Autodesk Fusion 360 part; units mm, degrees
note: some values were not read from the file. Chosen so that the rebuilt part matches the saved one: a direction. Set by a fixed rule: which sketch regions a step uses.
(part 4 of 6)
sketch "Sketch6" plane through (-0.4707, 0.1724, 6) normal (0, 0, 1) x (-0.999921, 0.012548, 0)
  arc A0 (-25.3686, -35.2487) -> (-25.5248, -36.2599) centre (-13.5, -37.5997) ccw
  arc A1 (-25.6343, -36.3483) -> (-25.5248, -36.2599) centre (-25.6242, -36.2488) ccw
  line L0 (-25.6343, -36.3483) -> (-26.119, -36.299)
  spline S0 degree 5 poles (-26.119, -36.299) (-26.1246, -36.2984) (-26.1359, -36.2974) (-26.1528, -36.2963) (-26.1754, -36.2957) (-26.2037, -36.2959) (-26.2321, -36.297) (-26.2605, -36.2985) (-26.2889, -36.3004) (-26.3173, -36.3024) (-26.3458, -36.3046) (-26.3743, -36.307) (-26.4028, -36.3098) (-26.4313, -36.313) (-26.4598, -36.3165) (-26.4883, -36.3204) (-26.5168, -36.3246) (-26.5454, -36.3291) (-26.5739, -36.3338) (-26.6025, -36.3387) (-26.6311, -36.3438) (-26.6596, -36.3492) (-26.6882, -36.3548) (-26.7168, -36.3606) (-26.7453, -36.3667) (-26.7739, -36.3729) (-26.8025, -36.3795) (-26.8311, -36.3862) (-26.8596, -36.3931) (-26.8882, -36.4002) (-26.9168, -36.4076) (-26.9453, -36.4151) (-26.9739, -36.4228) (-27.0024, -36.4307) (-27.031, -36.4388) (-27.0595, -36.4471) (-27.088, -36.4555) (-27.1166, -36.4642) (-27.1451, -36.473) (-27.1736, -36.482) (-27.2021, -36.4912) (-27.2306, -36.5006) (-27.2591, -36.5101) (-27.2875, -36.5198) (-27.316, -36.5297) (-27.3444, -36.5398) (-27.3729, -36.55) (-27.4013, -36.5604) (-27.4297, -36.5709) (-27.4581, -36.5816) (-27.4865, -36.5925) (-27.5149, -36.6035) (-27.5432, -36.6147) (-27.5716, -36.6261) (-27.5999, -36.6376) (-27.6282, -36.6493) (-27.6565, -36.6611) (-27.6848, -36.673) (-27.7131, -36.6852) (-27.7413, -36.6975) (-27.7696, -36.7099) (-27.7978, -36.7225) (-27.826, -36.7352) (-27.8541, -36.7481) (-27.8823, -36.7611) (-27.9104, -36.7743) (-27.9386, -36.7876) (-27.9666, -36.801) (-27.9947, -36.8146) (-28.0228, -36.8284) (-28.0508, -36.8423) (-28.0732, -36.8535) (-28.09, -36.862) (-28.1012, -36.8677) (-28.1068, -36.8705) knots 0 0 0 0 0 0 0.01428571 0.02857143 0.04285714 0.05714286 0.07142857 0.08571429 0.1 0.11428571 0.12857143 0.14285714 0.15714286 0.17142857 0.18571429 0.2 0.21428571 0.22857143 0.24285714 0.25714286 0.27142857 0.28571429 0.3 0.31428571 0.32857143 0.34285714 0.35714286 0.37142857 0.38571429 0.4 0.41428571 0.42857143 0.44285714 0.45714286 0.47142857 0.48571429 0.5 0.51428571 0.52857143 0.54285714 0.55714286 0.57142857 0.58571429 0.6 0.61428571 0.62857143 0.64285714 0.65714286 0.67142857 0.68571429 0.7 0.71428571 0.72857143 0.74285714 0.75714286 0.77142857 0.78571429 0.8 0.81428571 0.82857143 0.84285714 0.85714286 0.87142857 0.88571429 0.9 0.91428571 0.92857143 0.94285714 0.95714286 0.97142857 0.98571429 1 1 1 1 1 1
  arc A2 (-28.1068, -36.8705) -> (-28.1248, -37.6752) centre (-13.5, -37.5997) ccw
  spline S1 degree 5 poles (-28.1248, -37.6752) (-28.1193, -37.6783) (-28.1084, -37.6845) (-28.092, -37.6937) (-28.0701, -37.7059) (-28.0427, -37.7211) (-28.0153, -37.7361) (-27.9879, -37.7509) (-27.9604, -37.7656) (-27.9329, -37.7802) (-27.9054, -37.7946) (-27.8779, -37.8089) (-27.8503, -37.823) (-27.8227, -37.837) (-27.7951, -37.8508) (-27.7674, -37.8645) (-27.7398, -37.878) (-27.7121, -37.8914) (-27.6843, -37.9046) (-27.6566, -37.9177) (-27.6288, -37.9306) (-27.601, -37.9434) (-27.5732, -37.956) (-27.5454, -37.9684) (-27.5176, -37.9807) (-27.4897, -37.9928) (-27.4618, -38.0048) (-27.4339, -38.0166) (-27.4059, -38.0283) (-27.378, -38.0397) (-27.35, -38.051) (-27.322, -38.0622) (-27.294, -38.0732) (-27.266, -38.084) (-27.2379, -38.0946) (-27.2099, -38.105) (-27.1818, -38.1153) (-27.1537, -38.1254) (-27.1256, -38.1353) (-27.0975, -38.1451) (-27.0693, -38.1546) (-27.0412, -38.164) (-27.013, -38.1732) (-26.9848, -38.1822) (-26.9566, -38.1909) (-26.9284, -38.1995) (-26.9002, -38.2079) (-26.872, -38.2161) (-26.8437, -38.2241) (-26.8155, -38.2319) (-26.7872, -38.2395) (-26.7589, -38.2468) (-26.7307, -38.2539) (-26.7024, -38.2607) (-26.6741, -38.2674) (-26.6458, -38.2738) (-26.6175, -38.2799) (-26.5891, -38.2859) (-26.5608, -38.2917) (-26.5325, -38.2971) (-26.5042, -38.3023) (-26.4759, -38.3071) (-26.4475, -38.3116) (-26.4192, -38.3156) (-26.3908, -38.3193) (-26.3625, -38.3228) (-26.3342, -38.3261) (-26.3059, -38.3292) (-26.2776, -38.332) (-26.2493, -38.3343) (-26.221, -38.3358) (-26.1984, -38.3362) (-26.1815, -38.3359) (-26.1702, -38.3354) (-26.1645, -38.335) knots -1 -1 -1 -1 -1 -1 -0.98571429 -0.97142857 -0.95714286 -0.94285714 -0.92857143 -0.91428571 -0.9 -0.88571429 -0.87142857 -0.85714286 -0.84285714 -0.82857143 -0.81428571 -0.8 -0.78571429 -0.77142857 -0.75714286 -0.74285714 -0.72857143 -0.71428571 -0.7 -0.68571429 -0.67142857 -0.65714286 -0.64285714 -0.62857143 -0.61428571 -0.6 -0.58571429 -0.57142857 -0.55714286 -0.54285714 -0.52857143 -0.51428571 -0.5 -0.48571429 -0.47142857 -0.45714286 -0.44285714 -0.42857143 -0.41428571 -0.4 -0.38571429 -0.37142857 -0.35714286 -0.34285714 -0.32857143 -0.31428571 -0.3 -0.28571429 -0.27142857 -0.25714286 -0.24285714 -0.22857143 -0.21428571 -0.2 -0.18571429 -0.17142857 -0.15714286 -0.14285714 -0.12857143 -0.11428571 -0.1 -0.08571429 -0.07142857 -0.05714286 -0.04285714 -0.02857143 -0.01428571 0 0 0 0 0 0
  line L1 (-26.1645, -38.335) -> (-25.6781, -38.3074)
  arc A3 (-25.5727, -38.4007) -> (-25.6781, -38.3074) centre (-25.6724, -38.4073) ccw
  arc A4 (-25.5727, -38.4007) -> (-25.4618, -39.4178) centre (-13.5, -37.5997) ccw
  arc A5 (-25.5447, -39.5315) -> (-25.4618, -39.4178) centre (-25.5607, -39.4328) ccw
  line L2 (-25.5447, -39.5315) -> (-26.0257, -39.6094)
  spline S2 degree 5 poles (-26.0257, -39.6094) (-26.0312, -39.6103) (-26.0424, -39.6122) (-26.059, -39.6155) (-26.081, -39.6207) (-26.1083, -39.6283) (-26.1354, -39.6367) (-26.1624, -39.6455) (-26.1894, -39.6546) (-26.2164, -39.6639) (-26.2433, -39.6734) (-26.2702, -39.6832) (-26.297, -39.6932) (-26.3237, -39.7037) (-26.3503, -39.7145) (-26.3768, -39.7256) (-26.4033, -39.7371) (-26.4297, -39.7488) (-26.4561, -39.7607) (-26.4824, -39.7729) (-26.5087, -39.7852) (-26.5349, -39.7978) (-26.561, -39.8105) (-26.5871, -39.8236) (-26.6132, -39.8368) (-26.6391, -39.8503) (-26.665, -39.864) (-26.6909, -39.8779) (-26.7167, -39.892) (-26.7424, -39.9062) (-26.7681, -39.9207) (-26.7938, -39.9353) (-26.8194, -39.9502) (-26.8449, -39.9652) (-26.8704, -39.9804) (-26.8958, -39.9958) (-26.9212, -40.0114) (-26.9465, -40.0271) (-26.9717, -40.043) (-26.9969, -40.0591) (-27.0221, -40.0754) (-27.0472, -40.0918) (-27.0722, -40.1084) (-27.0972, -40.1251) (-27.1222, -40.142) (-27.147, -40.1591) (-27.1719, -40.1763) (-27.1966, -40.1937) (-27.2214, -40.2113) (-27.246, -40.2289) (-27.2706, -40.2468) (-27.2952, -40.2648) (-27.3197, -40.283) (-27.3441, -40.3013) (-27.3685, -40.3197) (-27.3928, -40.3383) (-27.4171, -40.357) (-27.4413, -40.3759) (-27.4655, -40.395) (-27.4896, -40.4141) (-27.5136, -40.4334) (-27.5376, -40.4529) (-27.5616, -40.4725) (-27.5855, -40.4922) (-27.6093, -40.5121) (-27.6331, -40.5321) (-27.6568, -40.5522) (-27.6804, -40.5725) (-27.704, -40.5929) (-27.7276, -40.6134) (-27.751, -40.6341) (-27.7698, -40.6508) (-27.7838, -40.6633) (-27.7932, -40.6717) (-27.7978, -40.6759) knots 0 0 0 0 0 0 0.01428571 0.02857143 0.04285714 0.05714286 0.07142857 0.08571429 0.1 0.11428571 0.12857143 0.14285714 0.15714286 0.17142857 0.18571429 0.2 0.21428571 0.22857143 0.24285714 0.25714286 0.27142857 0.28571429 0.3 0.31428571 0.32857143 0.34285714 0.35714286 0.37142857 0.38571429 0.4 0.41428571 0.42857143 0.44285714 0.45714286 0.47142857 0.48571429 0.5 0.51428571 0.52857143 0.54285714 0.55714286 0.57142857 0.58571429 0.6 0.61428571 0.62857143 0.64285714 0.65714286 0.67142857 0.68571429 0.7 0.71428571 0.72857143 0.74285714 0.75714286 0.77142857 0.78571429 0.8 0.81428571 0.82857143 0.84285714 0.85714286 0.87142857 0.88571429 0.9 0.91428571 0.92857143 0.94285714 0.95714286 0.97142857 0.98571429 1 1 1 1 1 1
  arc A6 (-27.7978, -40.6759) -> (-27.6069, -41.4578) centre (-13.5, -37.5997) ccw
  spline S3 degree 5 poles (-27.6069, -41.4578) (-27.6009, -41.4594) (-27.5887, -41.4625) (-27.5705, -41.4672) (-27.5462, -41.4734) (-27.5158, -41.4809) (-27.4854, -41.4883) (-27.4551, -41.4955) (-27.4248, -41.5026) (-27.3944, -41.5095) (-27.3641, -41.5163) (-27.3338, -41.523) (-27.3035, -41.5295) (-27.2733, -41.5359) (-27.243, -41.5421) (-27.2128, -41.5481) (-27.1825, -41.554) (-27.1523, -41.5598) (-27.1221, -41.5654) (-27.0919, -41.5708) (-27.0618, -41.5761) (-27.0316, -41.5813) (-27.0015, -41.5862) (-26.9714, -41.5911) (-26.9413, -41.5957) (-26.9112, -41.6002) (-26.8812, -41.6046) (-26.8512, -41.6088) (-26.8212, -41.6128) (-26.7912, -41.6166) (-26.7613, -41.6203) (-26.7314, -41.6238) (-26.7015, -41.6272) (-26.6716, -41.6304) (-26.6417, -41.6334) (-26.6119, -41.6362) (-26.5822, -41.6389) (-26.5524, -41.6413) (-26.5227, -41.6437) (-26.493, -41.6458) (-26.4633, -41.6477) (-26.4337, -41.6495) (-26.4041, -41.6511) (-26.3746, -41.6524) (-26.3451, -41.6536) (-26.3156, -41.6546) (-26.2862, -41.6554) (-26.2568, -41.656) (-26.2275, -41.6564) (-26.1981, -41.6567) (-26.1689, -41.6566) (-26.1397, -41.6564) (-26.1105, -41.6559) (-26.0814, -41.6552) (-26.0524, -41.6543) (-26.0234, -41.6532) (-25.9944, -41.6518) (-25.9655, -41.6503) (-25.9367, -41.6485) (-25.9079, -41.6464) (-25.8792, -41.6441) (-25.8506, -41.6414) (-25.8221, -41.6384) (-25.7937, -41.6349) (-25.7654, -41.6312) (-25.7371, -41.6272) (-25.7089, -41.6231) (-25.6807, -41.6187) (-25.6527, -41.6141) (-25.6247, -41.6091) (-25.597, -41.6032) (-25.5751, -41.5977) (-25.5588, -41.593) (-25.548, -41.5896) (-25.5427, -41.5878) knots -1 -1 -1 -1 -1 -1 -0.98571429 -0.97142857 -0.95714286 -0.94285714 -0.92857143 -0.91428571 -0.9 -0.88571429 -0.87142857 -0.85714286 -0.84285714 -0.82857143 -0.81428571 -0.8 -0.78571429 -0.77142857 -0.75714286 -0.74285714 -0.72857143 -0.71428571 -0.7 -0.68571429 -0.67142857 -0.65714286 -0.64285714 -0.62857143 -0.61428571 -0.6 -0.58571429 -0.57142857 -0.55714286 -0.54285714 -0.52857143 -0.51428571 -0.5 -0.48571429 -0.47142857 -0.45714286 -0.44285714 -0.42857143 -0.41428571 -0.4 -0.38571429 -0.37142857 -0.35714286 -0.34285714 -0.32857143 -0.31428571 -0.3 -0.28571429 -0.27142857 -0.25714286 -0.24285714 -0.22857143 -0.21428571 -0.2 -0.18571429 -0.17142857 -0.15714286 -0.14285714 -0.12857143 -0.11428571 -0.1 -0.08571429 -0.07142857 -0.05714286 -0.04285714 -0.02857143 -0.01428571 0 0 0 0 0 0
  line L3 (-25.5427, -41.5878) -> (-25.08, -41.4353)
  arc A7 (-24.954, -41.498) -> (-25.08, -41.4353) centre (-25.0487, -41.5302) ccw
  arc A8 (-24.954, -41.498) -> (-24.5837, -42.4518) centre (-13.5, -37.5997) ccw
  arc A9 (-24.6343, -42.5831) -> (-24.5837, -42.4518) centre (-24.6753, -42.4919) ccw
  line L4 (-24.6343, -42.5831) -> (-25.0787, -42.7828)
  spline S4 degree 5 poles (-25.0787, -42.7828) (-25.0839, -42.7851) (-25.0941, -42.7898) (-25.1093, -42.7974) (-25.1292, -42.8081) (-25.1536, -42.8225) (-25.1777, -42.8376) (-25.2015, -42.8531) (-25.2252, -42.8689) (-25.2488, -42.8849) (-25.2724, -42.901) (-25.2958, -42.9174) (-25.3191, -42.934) (-25.3422, -42.951) (-25.3651, -42.9683) (-25.3879, -42.986) (-25.4105, -43.0039) (-25.433, -43.022) (-25.4553, -43.0404) (-25.4776, -43.0589) (-25.4998, -43.0776) (-25.5218, -43.0965) (-25.5438, -43.1157) (-25.5656, -43.135) (-25.5873, -43.1545) (-25.6089, -43.1743) (-25.6304, -43.1942) (-25.6518, -43.2143) (-25.6731, -43.2346) (-25.6942, -43.255) (-25.7153, -43.2757) (-25.7363, -43.2964) (-25.7572, -43.3174) (-25.778, -43.3385) (-25.7986, -43.3598) (-25.8192, -43.3812) (-25.8397, -43.4028) (-25.86, -43.4246) (-25.8803, -43.4465) (-25.9005, -43.4686) (-25.9206, -43.4908) (-25.9406, -43.5131) (-25.9605, -43.5356) (-25.9803, -43.5583) (-26, -43.5811) (-26.0196, -43.604) (-26.0391, -43.6271) (-26.0586, -43.6503) (-26.0779, -43.6736) (-26.0971, -43.6971) (-26.1163, -43.7207) (-26.1353, -43.7444) (-26.1543, -43.7683) (-26.1732, -43.7923) (-26.192, -43.8164) (-26.2106, -43.8407) (-26.2292, -43.8651) (-26.2477, -43.8896) (-26.2662, -43.9142) (-26.2845, -43.939) (-26.3027, -43.9639) (-26.3209, -43.9889) (-26.3389, -44.014) (-26.3569, -44.0392) (-26.3747, -44.0646) (-26.3925, -44.0901) (-26.4102, -44.1157) (-26.4278, -44.1414) (-26.4453, -44.1672) (-26.4628, -44.1931) (-26.4801, -44.2192) (-26.4939, -44.2401) (-26.5042, -44.2558) (-26.511, -44.2664) (-26.5145, -44.2716) knots 0 0 0 0 0 0 0.01428571 0.02857143 0.04285714 0.05714286 0.07142857 0.08571429 0.1 0.11428571 0.12857143 0.14285714 0.15714286 0.17142857 0.18571429 0.2 0.21428571 0.22857143 0.24285714 0.25714286 0.27142857 0.28571429 0.3 0.31428571 0.32857143 0.34285714 0.35714286 0.37142857 0.38571429 0.4 0.41428571 0.42857143 0.44285714 0.45714286 0.47142857 0.48571429 0.5 0.51428571 0.52857143 0.54285714 0.55714286 0.57142857 0.58571429 0.6 0.61428571 0.62857143 0.64285714 0.65714286 0.67142857 0.68571429 0.7 0.71428571 0.72857143 0.74285714 0.75714286 0.77142857 0.78571429 0.8 0.81428571 0.82857143 0.84285714 0.85714286 0.87142857 0.88571429 0.9 0.91428571 0.92857143 0.94285714 0.95714286 0.97142857 0.98571429 1 1 1 1 1 1
  arc A10 (-26.5145, -44.2716) -> (-26.1277, -44.9775) centre (-13.5, -37.5997) ccw
  spline S5 degree 5 poles (-26.1277, -44.9775) (-26.1214, -44.9775) (-26.1089, -44.9773) (-26.09, -44.9771) (-26.065, -44.9768) (-26.0337, -44.9762) (-26.0025, -44.9755) (-25.9713, -44.9746) (-25.9401, -44.9736) (-25.9091, -44.9725) (-25.878, -44.9712) (-25.847, -44.9698) (-25.8161, -44.9682) (-25.7852, -44.9665) (-25.7544, -44.9647) (-25.7236, -44.9627) (-25.6928, -44.9606) (-25.6622, -44.9583) (-25.6316, -44.9559) (-25.601, -44.9534) (-25.5705, -44.9507) (-25.54, -44.9478) (-25.5097, -44.9449) (-25.4793, -44.9417) (-25.4491, -44.9384) (-25.4189, -44.935) (-25.3887, -44.9314) (-25.3586, -44.9277) (-25.3286, -44.9238) (-25.2987, -44.9198) (-25.2688, -44.9156) (-25.239, -44.9112) (-25.2092, -44.9067) (-25.1796, -44.9021) (-25.15, -44.8973) (-25.1204, -44.8923) (-25.091, -44.8871) (-25.0616, -44.8818) (-25.0323, -44.8764) (-25.0031, -44.8708) (-24.9739, -44.865) (-24.9449, -44.859) (-24.9159, -44.8528) (-24.887, -44.8465) (-24.8582, -44.84) (-24.8295, -44.8334) (-24.8008, -44.8265) (-24.7723, -44.8195) (-24.7438, -44.8123) (-24.7155, -44.8049) (-24.6872, -44.7974) (-24.659, -44.7896) (-24.631, -44.7816) (-24.6031, -44.7734) (-24.5753, -44.765) (-24.5476, -44.7563) (-24.5199, -44.7475) (-24.4924, -44.7386) (-24.465, -44.7294) (-24.4378, -44.72) (-24.4107, -44.7103) (-24.3837, -44.7003) (-24.357, -44.6899) (-24.3304, -44.6793) (-24.304, -44.6683) (-24.2777, -44.6572) (-24.2516, -44.6459) (-24.2255, -44.6344) (-24.1996, -44.6227) (-24.1739, -44.6106) (-24.1487, -44.5977) (-24.1289, -44.5867) (-24.1144, -44.578) (-24.1049, -44.5719) (-24.1001, -44.5688) knots -1 -1 -1 -1 -1 -1 -0.98571429 -0.97142857 -0.95714286 -0.94285714 -0.92857143 -0.91428571 -0.9 -0.88571429 -0.87142857 -0.85714286 -0.84285714 -0.82857143 -0.81428571 -0.8 -0.78571429 -0.77142857 -0.75714286 -0.74285714 -0.72857143 -0.71428571 -0.7 -0.68571429 -0.67142857 -0.65714286 -0.64285714 -0.62857143 -0.61428571 -0.6 -0.58571429 -0.57142857 -0.55714286 -0.54285714 -0.52857143 -0.51428571 -0.5 -0.48571429 -0.47142857 -0.45714286 -0.44285714 -0.42857143 -0.41428571 -0.4 -0.38571429 -0.37142857 -0.35714286 -0.34285714 -0.32857143 -0.31428571 -0.3 -0.28571429 -0.27142857 -0.25714286 -0.24285714 -0.22857143 -0.21428571 -0.2 -0.18571429 -0.17142857 -0.15714286 -0.14285714 -0.12857143 -0.11428571 -0.1 -0.08571429 -0.07142857 -0.05714286 -0.04285714 -0.02857143 -0.01428571 0 0 0 0 0 0
  line L5 (-24.1001, -44.5688) -> (-23.6927, -44.3017)
  arc A11 (-23.5548, -44.3297) -> (-23.6927, -44.3017) centre (-23.6379, -44.3853) ccw
  arc A12 (-23.5548, -44.3297) -> (-22.9502, -45.1551) centre (-13.5, -37.5997) ccw
  arc A13 (-22.9651, -45.2951) -> (-22.9502, -45.1551) centre (-23.0283, -45.2176) ccw
  line L6 (-22.9651, -45.2951) -> (-23.3427, -45.603)
  spline S6 degree 5 poles (-23.3427, -45.603) (-23.3471, -45.6065) (-23.3558, -45.6138) (-23.3685, -45.625) (-23.385, -45.6405) (-23.4048, -45.6607) (-23.4241, -45.6815) (-23.4431, -45.7027) (-23.4619, -45.724) (-23.4806, -45.7456) (-23.4991, -45.7673) (-23.5175, -45.7891) (-23.5357, -45.8112) (-23.5536, -45.8336) (-23.5713, -45.8563) (-23.5887, -45.8792) (-23.6059, -45.9024) (-23.6229, -45.9257) (-23.6398, -45.9492) (-23.6565, -45.9729) (-23.6731, -45.9967) (-23.6895, -46.0207) (-23.7058, -46.0449) (-23.7219, -46.0692) (-23.7378, -46.0937) (-23.7535, -46.1183) (-23.7691, -46.1431) (-23.7846, -46.1681) (-23.7999, -46.1932) (-23.815, -46.2184) (-23.8301, -46.2438) (-23.8449, -46.2693) (-23.8597, -46.295) (-23.8743, -46.3207) (-23.8887, -46.3466) (-23.9031, -46.3727) (-23.9172, -46.3988) (-23.9313, -46.4251) (-23.9452, -46.4516) (-23.959, -46.4781) (-23.9727, -46.5047) (-23.9862, -46.5315) (-23.9996, -46.5584) (-24.0128, -46.5854) (-24.026, -46.6125) (-24.039, -46.6397) (-24.0519, -46.6671) (-24.0646, -46.6945) (-24.0773, -46.722) (-24.0898, -46.7497) (-24.1022, -46.7775) (-24.1144, -46.8053) (-24.1266, -46.8333) (-24.1386, -46.8614) (-24.1505, -46.8895) (-24.1622, -46.9178) (-24.1739, -46.9462) (-24.1854, -46.9746) (-24.1968, -47.0032) (-24.2081, -47.0319) (-24.2193, -47.0606) (-24.2304, -47.0895) (-24.2413, -47.1184) (-24.2521, -47.1474) (-24.2628, -47.1765) (-24.2734, -47.2057) (-24.2839, -47.235) (-24.2942, -47.2644) (-24.3044, -47.2939) (-24.3146, -47.3235) (-24.3246, -47.3531) (-24.3325, -47.3769) (-24.3383, -47.3948) (-24.3422, -47.4067) (-24.3442, -47.4127) knots 0 0 0 0 0 0 0.01428571 0.02857143 0.04285714 0.05714286 0.07142857 0.08571429 0.1 0.11428571 0.12857143 0.14285714 0.15714286 0.17142857 0.18571429 0.2 0.21428571 0.22857143 0.24285714 0.25714286 0.27142857 0.28571429 0.3 0.31428571 0.32857143 0.34285714 0.35714286 0.37142857 0.38571429 0.4 0.41428571 0.42857143 0.44285714 0.45714286 0.47142857 0.48571429 0.5 0.51428571 0.52857143 0.54285714 0.55714286 0.57142857 0.58571429 0.6 0.61428571 0.62857143 0.64285714 0.65714286 0.67142857 0.68571429 0.7 0.71428571 0.72857143 0.74285714 0.75714286 0.77142857 0.78571429 0.8 0.81428571 0.82857143 0.84285714 0.85714286 0.87142857 0.88571429 0.9 0.91428571 0.92857143 0.94285714 0.95714286 0.97142857 0.98571429 1 1 1 1 1 1
  arc A14 (-24.3442, -47.4127) -> (-23.7879, -47.9944) centre (-13.5, -37.5997) ccw
  spline S7 degree 5 poles (-23.7879, -47.9944) (-23.7819, -47.9927) (-23.7698, -47.9894) (-23.7516, -47.9843) (-23.7275, -47.9775) (-23.6975, -47.9688) (-23.6675, -47.96) (-23.6376, -47.9511) (-23.6078, -47.9421) (-23.578, -47.9329) (-23.5484, -47.9237) (-23.5188, -47.9143) (-23.4893, -47.9048) (-23.4599, -47.8951) (-23.4306, -47.8854) (-23.4014, -47.8755) (-23.3723, -47.8655) (-23.3432, -47.8554) (-23.3143, -47.8451) (-23.2854, -47.8348) (-23.2566, -47.8243) (-23.228, -47.8137) (-23.1994, -47.8029) (-23.1709, -47.792) (-23.1425, -47.781) (-23.1142, -47.7699) (-23.086, -47.7586) (-23.0579, -47.7472) (-23.03, -47.7357) (-23.0021, -47.7241) (-22.9743, -47.7123) (-22.9466, -47.7004) (-22.9191, -47.6883) (-22.8916, -47.6762) (-22.8643, -47.6638) (-22.837, -47.6514) (-22.8099, -47.6388) (-22.7829, -47.6261) (-22.756, -47.6132) (-22.7292, -47.6002) (-22.7026, -47.5871) (-22.676, -47.5738) (-22.6496, -47.5604) (-22.6234, -47.5468) (-22.5972, -47.533) (-22.5712, -47.5192) (-22.5453, -47.5052) (-22.5196, -47.491) (-22.4939, -47.4767) (-22.4684, -47.4622) (-22.4431, -47.4476) (-22.4179, -47.4328) (-22.3929, -47.4178) (-22.3681, -47.4026) (-22.3434, -47.3873) (-22.3188, -47.3718) (-22.2945, -47.3562) (-22.2702, -47.3404) (-22.2461, -47.3244) (-22.2222, -47.3082) (-22.1985, -47.2919) (-22.1751, -47.2752) (-22.1519, -47.2583) (-22.129, -47.2412) (-22.1064, -47.2238) (-22.0839, -47.2062) (-22.0615, -47.1885) (-22.0393, -47.1707) (-22.0173, -47.1526) (-21.9957, -47.1343) (-21.9746, -47.1154) (-21.9584, -47.0996) (-21.9466, -47.0874) (-21.939, -47.0791) (-21.9352, -47.0748) knots -1 -1 -1 -1 -1 -1 -0.98571429 -0.97142857 -0.95714286 -0.94285714 -0.92857143 -0.91428571 -0.9 -0.88571429 -0.87142857 -0.85714286 -0.84285714 -0.82857143 -0.81428571 -0.8 -0.78571429 -0.77142857 -0.75714286 -0.74285714 -0.72857143 -0.71428571 -0.7 -0.68571429 -0.67142857 -0.65714286 -0.64285714 -0.62857143 -0.61428571 -0.6 -0.58571429 -0.57142857 -0.55714286 -0.54285714 -0.52857143 -0.51428571 -0.5 -0.48571429 -0.47142857 -0.45714286 -0.44285714 -0.42857143 -0.41428571 -0.4 -0.38571429 -0.37142857 -0.35714286 -0.34285714 -0.32857143 -0.31428571 -0.3 -0.28571429 -0.27142857 -0.25714286 -0.24285714 -0.22857143 -0.21428571 -0.2 -0.18571429 -0.17142857 -0.15714286 -0.14285714 -0.12857143 -0.11428571 -0.1 -0.08571429 -0.07142857 -0.05714286 -0.04285714 -0.02857143 -0.01428571 0 0 0 0 0 0
  line L7 (-21.9352, -47.0748) -> (-21.6108, -46.7114)
  arc A15 (-21.4703, -46.7027) -> (-21.6108, -46.7114) centre (-21.5362, -46.778) ccw
  arc A16 (-21.4703, -46.7027) -> (-20.6727, -47.3436) centre (-13.5, -37.5997) ccw
  arc A17 (-20.6509, -47.4826) -> (-20.6727, -47.3436) centre (-20.732, -47.4241) ccw
  line L8 (-20.6509, -47.4826) -> (-20.9359, -47.8777)
  spline S8 degree 5 poles (-20.9359, -47.8777) (-20.9393, -47.8823) (-20.9458, -47.8916) (-20.9552, -47.9057) (-20.967, -47.9249) (-20.981, -47.9496) (-20.9942, -47.9747) (-21.0071, -48) (-21.0197, -48.0255) (-21.0322, -48.0512) (-21.0445, -48.0769) (-21.0566, -48.1028) (-21.0685, -48.1289) (-21.08, -48.1551) (-21.0912, -48.1816) (-21.1021, -48.2083) (-21.1127, -48.2351) (-21.1231, -48.262) (-21.1333, -48.2891) (-21.1433, -48.3163) (-21.1532, -48.3436) (-21.1628, -48.371) (-21.1723, -48.3986) (-21.1815, -48.4262) (-21.1905, -48.454) (-21.1994, -48.4819) (-21.208, -48.5099) (-21.2165, -48.538) (-21.2248, -48.5662) (-21.2329, -48.5945) (-21.2408, -48.6229) (-21.2486, -48.6514) (-21.2562, -48.68) (-21.2636, -48.7086) (-21.2709, -48.7374) (-21.278, -48.7663) (-21.2849, -48.7952) (-21.2917, -48.8242) (-21.2983, -48.8534) (-21.3047, -48.8826) (-21.311, -48.9118) (-21.3172, -48.9412) (-21.3231, -48.9706) (-21.329, -49.0001) (-21.3346, -49.0297) (-21.3402, -49.0594) (-21.3455, -49.0891) (-21.3508, -49.1189) (-21.3558, -49.1488) (-21.3607, -49.1788) (-21.3655, -49.2088) (-21.3702, -49.2389) (-21.3746, -49.269) (-21.379, -49.2993) (-21.3832, -49.3295) (-21.3872, -49.3599) (-21.3912, -49.3903) (-21.3949, -49.4208) (-21.3986, -49.4513) (-21.402, -49.4819) (-21.4054, -49.5126) (-21.4086, -49.5433) (-21.4117, -49.5741) (-21.4146, -49.6049) (-21.4174, -49.6358) (-21.4201, -49.6668) (-21.4226, -49.6978) (-21.425, -49.7289) (-21.4273, -49.76) (-21.4294, -49.7912) (-21.4314, -49.8224) (-21.4328, -49.8474) (-21.4339, -49.8662) (-21.4346, -49.8787) (-21.4349, -49.885) knots 0 0 0 0 0 0 0.01428571 0.02857143 0.04285714 0.05714286 0.07142857 0.08571429 0.1 0.11428571 0.12857143 0.14285714 0.15714286 0.17142857 0.18571429 0.2 0.21428571 0.22857143 0.24285714 0.25714286 0.27142857 0.28571429 0.3 0.31428571 0.32857143 0.34285714 0.35714286 0.37142857 0.38571429 0.4 0.41428571 0.42857143 0.44285714 0.45714286 0.47142857 0.48571429 0.5 0.51428571 0.52857143 0.54285714 0.55714286 0.57142857 0.58571429 0.6 0.61428571 0.62857143 0.64285714 0.65714286 0.67142857 0.68571429 0.7 0.71428571 0.72857143 0.74285714 0.75714286 0.77142857 0.78571429 0.8 0.81428571 0.82857143 0.84285714 0.85714286 0.87142857 0.88571429 0.9 0.91428571 0.92857143 0.94285714 0.95714286 0.97142857 0.98571429 1 1 1 1 1 1
  arc A18 (-21.4349, -49.885) -> (-20.747, -50.3029) centre (-13.5, -37.5997) ccw
  spline S9 degree 5 poles (-20.747, -50.3029) (-20.7416, -50.2997) (-20.7308, -50.2934) (-20.7146, -50.2838) (-20.6931, -50.2709) (-20.6663, -50.2548) (-20.6396, -50.2385) (-20.613, -50.2222) (-20.5865, -50.2058) (-20.5602, -50.1892) (-20.5339, -50.1726) (-20.5078, -50.1559) (-20.4818, -50.1391) (-20.4559, -50.1222) (-20.4301, -50.1051) (-20.4044, -50.088) (-20.3789, -50.0708) (-20.3534, -50.0535) (-20.3281, -50.0362) (-20.3029, -50.0187) (-20.2779, -50.0011) (-20.2529, -49.9834) (-20.2281, -49.9656) (-20.2034, -49.9477) (-20.1788, -49.9298) (-20.1544, -49.9117) (-20.1301, -49.8935) (-20.1059, -49.8753) (-20.0818, -49.8569) (-20.0579, -49.8384) (-20.0341, -49.8198) (-20.0105, -49.8012) (-19.987, -49.7824) (-19.9636, -49.7635) (-19.9404, -49.7446) (-19.9173, -49.7255) (-19.8944, -49.7063) (-19.8716, -49.687) (-19.8489, -49.6676) (-19.8264, -49.6482) (-19.8041, -49.6286) (-19.7819, -49.6089) (-19.7599, -49.5891) (-19.738, -49.5691) (-19.7163, -49.5491) (-19.6948, -49.529) (-19.6734, -49.5087) (-19.6522, -49.4884) (-19.6311, -49.4679) (-19.6103, -49.4473) (-19.5896, -49.4267) (-19.5691, -49.4058) (-19.5488, -49.3849) (-19.5287, -49.3638) (-19.5088, -49.3426) (-19.4891, -49.3213) (-19.4696, -49.2999) (-19.4503, -49.2784) (-19.4312, -49.2567) (-19.4123, -49.2349) (-19.3936, -49.213) (-19.3753, -49.1908) (-19.3573, -49.1685) (-19.3396, -49.146) (-19.3222, -49.1233) (-19.305, -49.1005) (-19.288, -49.0776) (-19.2712, -49.0547) (-19.2546, -49.0316) (-19.2385, -49.0082) (-19.223, -48.9845) (-19.2114, -48.9651) (-19.2032, -48.9503) (-19.198, -48.9402) (-19.1955, -48.9352) knots -1 -1 -1 -1 -1 -1 -0.98571429 -0.97142857 -0.95714286 -0.94285714 -0.92857143 -0.91428571 -0.9 -0.88571429 -0.87142857 -0.85714286 -0.84285714 -0.82857143 -0.81428571 -0.8 -0.78571429 -0.77142857 -0.75714286 -0.74285714 -0.72857143 -0.71428571 -0.7 -0.68571429 -0.67142857 -0.65714286 -0.64285714 -0.62857143 -0.61428571 -0.6 -0.58571429 -0.57142857 -0.55714286 -0.54285714 -0.52857143 -0.51428571 -0.5 -0.48571429 -0.47142857 -0.45714286 -0.44285714 -0.42857143 -0.41428571 -0.4 -0.38571429 -0.37142857 -0.35714286 -0.34285714 -0.32857143 -0.31428571 -0.3 -0.28571429 -0.27142857 -0.25714286 -0.24285714 -0.22857143 -0.21428571 -0.2 -0.18571429 -0.17142857 -0.15714286 -0.14285714 -0.12857143 -0.11428571 -0.1 -0.08571429 -0.07142857 -0.05714286 -0.04285714 -0.02857143 -0.01428571 0 0 0 0 0 0
  line L9 (-19.1955, -48.9352) -> (-18.9761, -48.5001)
  arc A19 (-18.8427, -48.4554) -> (-18.9761, -48.5001) centre (-18.8868, -48.5451) ccw
  arc A20 (-18.8427, -48.4554) -> (-17.9064, -48.868) centre (-13.5, -37.5997) ccw
  arc A21 (-17.8493, -48.9967) -> (-17.9064, -48.868) centre (-17.9428, -48.9611) ccw
  line L10 (-17.8493, -48.9967) -> (-18.0224, -49.4521)
  spline S10 degree 5 poles (-18.0224, -49.4521) (-18.0244, -49.4574) (-18.0283, -49.468) (-18.0338, -49.484) (-18.0402, -49.5057) (-18.0473, -49.5331) (-18.0537, -49.5608) (-18.0595, -49.5886) (-18.0651, -49.6165) (-18.0705, -49.6445) (-18.0757, -49.6726) (-18.0807, -49.7007) (-18.0854, -49.729) (-18.0898, -49.7573) (-18.0937, -49.7858) (-18.0973, -49.8143) (-18.1007, -49.843) (-18.1037, -49.8717) (-18.1066, -49.9005) (-18.1092, -49.9294) (-18.1117, -49.9583) (-18.1139, -49.9873) (-18.1159, -50.0163) (-18.1177, -50.0454) (-18.1192, -50.0746) (-18.1205, -50.1038) (-18.1216, -50.1331) (-18.1225, -50.1624) (-18.1232, -50.1918) (-18.1237, -50.2213) (-18.124, -50.2507) (-18.1242, -50.2803) (-18.1241, -50.3099) (-18.1239, -50.3395) (-18.1235, -50.3691) (-18.1228, -50.3989) (-18.122, -50.4286) (-18.1211, -50.4584) (-18.1199, -50.4882) (-18.1186, -50.5181) (-18.1171, -50.548) (-18.1154, -50.578) (-18.1136, -50.6079) (-18.1116, -50.638) (-18.1094, -50.668) (-18.107, -50.6981) (-18.1045, -50.7282) (-18.1019, -50.7583) (-18.099, -50.7885) (-18.096, -50.8187) (-18.0929, -50.849) (-18.0896, -50.8792) (-18.0861, -50.9095) (-18.0825, -50.9398) (-18.0787, -50.9702) (-18.0747, -51.0005) (-18.0706, -51.0309) (-18.0664, -51.0614) (-18.062, -51.0918) (-18.0574, -51.1223) (-18.0527, -51.1527) (-18.0479, -51.1833) (-18.0429, -51.2138) (-18.0378, -51.2443) (-18.0325, -51.2749) (-18.027, -51.3055) (-18.0214, -51.3361) (-18.0157, -51.3667) (-18.0098, -51.3974) (-18.0038, -51.428) (-17.9976, -51.4587) (-17.9926, -51.4832) (-17.9888, -51.5017) (-17.9862, -51.5139) (-17.9849, -51.5201) knots 0 0 0 0 0 0 0.01428571 0.02857143 0.04285714 0.05714286 0.07142857 0.08571429 0.1 0.11428571 0.12857143 0.14285714 0.15714286 0.17142857 0.18571429 0.2 0.21428571 0.22857143 0.24285714 0.25714286 0.27142857 0.28571429 0.3 0.31428571 0.32857143 0.34285714 0.35714286 0.37142857 0.38571429 0.4 0.41428571 0.42857143 0.44285714 0.45714286 0.47142857 0.48571429 0.5 0.51428571 0.52857143 0.54285714 0.55714286 0.57142857 0.58571429 0.6 0.61428571 0.62857143 0.64285714 0.65714286 0.67142857 0.68571429 0.7 0.71428571 0.72857143 0.74285714 0.75714286 0.77142857 0.78571429 0.8 0.81428571 0.82857143 0.84285714 0.85714286 0.87142857 0.88571429 0.9 0.91428571 0.92857143 0.94285714 0.95714286 0.97142857 0.98571429 1 1 1 1 1 1
  arc A22 (-17.9849, -51.5201) -> (-17.2122, -51.7457) centre (-13.5, -37.5997) ccw
  spline S11 degree 5 poles (-17.2122, -51.7457) (-17.2078, -51.7413) (-17.199, -51.7323) (-17.1859, -51.7188) (-17.1684, -51.7009) (-17.1467, -51.6783) (-17.1251, -51.6557) (-17.1037, -51.6331) (-17.0824, -51.6103) (-17.0612, -51.5876) (-17.0402, -51.5647) (-17.0192, -51.5418) (-16.9985, -51.5188) (-16.9778, -51.4958) (-16.9573, -51.4727) (-16.937, -51.4495) (-16.9167, -51.4263) (-16.8966, -51.403) (-16.8767, -51.3796) (-16.8569, -51.3562) (-16.8372, -51.3328) (-16.8177, -51.3092) (-16.7983, -51.2856) (-16.7791, -51.262) (-16.76, -51.2382) (-16.7411, -51.2145) (-16.7223, -51.1906) (-16.7037, -51.1667) (-16.6852, -51.1427) (-16.6669, -51.1187) (-16.6487, -51.0946) (-16.6307, -51.0705) (-16.6128, -51.0462) (-16.5952, -51.022) (-16.5776, -50.9976) (-16.5603, -50.9732) (-16.5431, -50.9488) (-16.526, -50.9242) (-16.5092, -50.8997) (-16.4925, -50.875) (-16.476, -50.8503) (-16.4597, -50.8255) (-16.4435, -50.8007) (-16.4275, -50.7758) (-16.4118, -50.7508) (-16.3962, -50.7258) (-16.3808, -50.7007) (-16.3655, -50.6756) (-16.3505, -50.6504) (-16.3357, -50.6251) (-16.321, -50.5998) (-16.3066, -50.5743) (-16.2925, -50.5489) (-16.2785, -50.5233) (-16.2648, -50.4977) (-16.2513, -50.472) (-16.238, -50.4463) (-16.2249, -50.4205) (-16.212, -50.3946) (-16.1994, -50.3687) (-16.1871, -50.3426) (-16.1751, -50.3165) (-16.1635, -50.2903) (-16.1522, -50.264) (-16.1413, -50.2376) (-16.1306, -50.2111) (-16.1201, -50.1846) (-16.1098, -50.1581) (-16.0997, -50.1314) (-16.0902, -50.1047) (-16.0814, -50.0778) (-16.0752, -50.0561) (-16.0712, -50.0396) (-16.0687, -50.0286) (-16.0676, -50.023) knots -1 -1 -1 -1 -1 -1 -0.98571429 -0.97142857 -0.95714286 -0.94285714 -0.92857143 -0.91428571 -0.9 -0.88571429 -0.87142857 -0.85714286 -0.84285714 -0.82857143 -0.81428571 -0.8 -0.78571429 -0.77142857 -0.75714286 -0.74285714 -0.72857143 -0.71428571 -0.7 -0.68571429 -0.67142857 -0.65714286 -0.64285714 -0.62857143 -0.61428571 -0.6 -0.58571429 -0.57142857 -0.55714286 -0.54285714 -0.52857143 -0.51428571 -0.5 -0.48571429 -0.47142857 -0.45714286 -0.44285714 -0.42857143 -0.41428571 -0.4 -0.38571429 -0.37142857 -0.35714286 -0.34285714 -0.32857143 -0.31428571 -0.3 -0.28571429 -0.27142857 -0.25714286 -0.24285714 -0.22857143 -0.21428571 -0.2 -0.18571429 -0.17142857 -0.15714286 -0.14285714 -0.12857143 -0.11428571 -0.1 -0.08571429 -0.07142857 -0.05714286 -0.04285714 -0.02857143 -0.01428571 0 0 0 0 0 0
  line L11 (-16.0676, -50.023) -> (-15.9683, -49.546)
  arc A23 (-15.851, -49.4683) -> (-15.9683, -49.546) centre (-15.8704, -49.5664) ccw
  arc A24 (-15.851, -49.4683) -> (-14.8398, -49.6245) centre (-13.5, -37.5997) ccw
  arc A25 (-14.7514, -49.734) -> (-14.8398, -49.6245) centre (-14.8509, -49.7239) ccw
  line L12 (-14.7514, -49.734) -> (-14.8007, -50.2187)
  spline S12 degree 5 poles (-14.8007, -50.2187) (-14.8013, -50.2243) (-14.8023, -50.2356) (-14.8034, -50.2525) (-14.804, -50.2751) (-14.8038, -50.3034) (-14.8027, -50.3318) (-14.8012, -50.3602) (-14.7994, -50.3886) (-14.7973, -50.4171) (-14.7951, -50.4455) (-14.7927, -50.474) (-14.7899, -50.5025) (-14.7868, -50.531) (-14.7832, -50.5595) (-14.7793, -50.588) (-14.7751, -50.6166) (-14.7706, -50.6451) (-14.7659, -50.6737) (-14.761, -50.7022) (-14.7559, -50.7308) (-14.7505, -50.7593) (-14.7449, -50.7879) (-14.7391, -50.8165) (-14.7331, -50.8451) (-14.7268, -50.8736) (-14.7203, -50.9022) (-14.7135, -50.9308) (-14.7066, -50.9593) (-14.6995, -50.9879) (-14.6922, -51.0165) (-14.6846, -51.045) (-14.6769, -51.0736) (-14.669, -51.1021) (-14.6609, -51.1307) (-14.6527, -51.1592) (-14.6442, -51.1877) (-14.6355, -51.2163) (-14.6267, -51.2448) (-14.6177, -51.2733) (-14.6085, -51.3018) (-14.5991, -51.3303) (-14.5896, -51.3588) (-14.5799, -51.3872) (-14.57, -51.4157) (-14.5599, -51.4442) (-14.5497, -51.4726) (-14.5393, -51.501) (-14.5288, -51.5294) (-14.5181, -51.5578) (-14.5072, -51.5862) (-14.4962, -51.6146) (-14.485, -51.643) (-14.4736, -51.6713) (-14.4621, -51.6996) (-14.4505, -51.7279) (-14.4386, -51.7562) (-14.4267, -51.7845) (-14.4145, -51.8128) (-14.4023, -51.841) (-14.3898, -51.8693) (-14.3773, -51.8975) (-14.3645, -51.9257) (-14.3516, -51.9539) (-14.3386, -51.982) (-14.3255, -52.0102) (-14.3121, -52.0383) (-14.2987, -52.0664) (-14.2851, -52.0944) (-14.2713, -52.1225) (-14.2574, -52.1505) (-14.2462, -52.1729) (-14.2377, -52.1897) (-14.232, -52.2009) (-14.2292, -52.2065) knots 0 0 0 0 0 0 0.01428571 0.02857143 0.04285714 0.05714286 0.07142857 0.08571429 0.1 0.11428571 0.12857143 0.14285714 0.15714286 0.17142857 0.18571429 0.2 0.21428571 0.22857143 0.24285714 0.25714286 0.27142857 0.28571429 0.3 0.31428571 0.32857143 0.34285714 0.35714286 0.37142857 0.38571429 0.4 0.41428571 0.42857143 0.44285714 0.45714286 0.47142857 0.48571429 0.5 0.51428571 0.52857143 0.54285714 0.55714286 0.57142857 0.58571429 0.6 0.61428571 0.62857143 0.64285714 0.65714286 0.67142857 0.68571429 0.7 0.71428571 0.72857143 0.74285714 0.75714286 0.77142857 0.78571429 0.8 0.81428571 0.82857143 0.84285714 0.85714286 0.87142857 0.88571429 0.9 0.91428571 0.92857143 0.94285714 0.95714286 0.97142857 0.98571429 1 1 1 1 1 1
  arc A26 (-14.2292, -52.2065) -> (-13.4245, -52.2245) centre (-13.5, -37.5997) ccw
  spline S13 degree 5 poles (-13.4245, -52.2245) (-13.4214, -52.2191) (-13.4152, -52.2081) (-13.406, -52.1917) (-13.3938, -52.1698) (-13.3786, -52.1425) (-13.3637, -52.115) (-13.3488, -52.0876) (-13.3341, -52.0601) (-13.3195, -52.0326) (-13.3051, -52.0051) (-13.2909, -51.9776) (-13.2767, -51.95) (-13.2628, -51.9224) (-13.2489, -51.8948) (-13.2352, -51.8671) (-13.2217, -51.8395) (-13.2083, -51.8118) (-13.1951, -51.7841) (-13.182, -51.7563) (-13.1691, -51.7285) (-13.1564, -51.7008) (-13.1438, -51.673) (-13.1313, -51.6451) (-13.119, -51.6173) (-13.1069, -51.5894) (-13.0949, -51.5615) (-13.0831, -51.5336) (-13.0715, -51.5057) (-13.06, -51.4777) (-13.0487, -51.4497) (-13.0375, -51.4217) (-13.0266, -51.3937) (-13.0158, -51.3657) (-13.0051, -51.3377) (-12.9947, -51.3096) (-12.9844, -51.2815) (-12.9743, -51.2534) (-12.9644, -51.2253) (-12.9546, -51.1972) (-12.9451, -51.169) (-12.9357, -51.1409) (-12.9265, -51.1127) (-12.9176, -51.0845) (-12.9088, -51.0563) (-12.9002, -51.0281) (-12.8918, -50.9999) (-12.8836, -50.9717) (-12.8756, -50.9434) (-12.8678, -50.9152) (-12.8603, -50.8869) (-12.8529, -50.8587) (-12.8458, -50.8304) (-12.839, -50.8021) (-12.8324, -50.7738) (-12.826, -50.7455) (-12.8198, -50.7172) (-12.8138, -50.6889) (-12.8081, -50.6605) (-12.8026, -50.6322) (-12.7974, -50.6039) (-12.7926, -50.5756) (-12.7882, -50.5472) (-12.7841, -50.5189) (-12.7804, -50.4906) (-12.7769, -50.4622) (-12.7736, -50.4339) (-12.7705, -50.4056) (-12.7677, -50.3773) (-12.7654, -50.349) (-12.7639, -50.3207) (-12.7635, -50.2981) (-12.7639, -50.2812) (-12.7644, -50.2699) (-12.7647, -50.2642) knots -1 -1 -1 -1 -1 -1 -0.98571429 -0.97142857 -0.95714286 -0.94285714 -0.92857143 -0.91428571 -0.9 -0.88571429 -0.87142857 -0.85714286 -0.84285714 -0.82857143 -0.81428571 -0.8 -0.78571429 -0.77142857 -0.75714286 -0.74285714 -0.72857143 -0.71428571 -0.7 -0.68571429 -0.67142857 -0.65714286 -0.64285714 -0.62857143 -0.61428571 -0.6 -0.58571429 -0.57142857 -0.55714286 -0.54285714 -0.52857143 -0.51428571 -0.5 -0.48571429 -0.47142857 -0.45714286 -0.44285714 -0.42857143 -0.41428571 -0.4 -0.38571429 -0.37142857 -0.35714286 -0.34285714 -0.32857143 -0.31428571 -0.3 -0.28571429 -0.27142857 -0.25714286 -0.24285714 -0.22857143 -0.21428571 -0.2 -0.18571429 -0.17142857 -0.15714286 -0.14285714 -0.12857143 -0.11428571 -0.1 -0.08571429 -0.07142857 -0.05714286 -0.04285714 -0.02857143 -0.01428571 0 0 0 0 0 0
  line L13 (-12.7647, -50.2642) -> (-12.7923, -49.7778)
  arc A27 (-12.6991, -49.6724) -> (-12.7923, -49.7778) centre (-12.6924, -49.7722) ccw
  arc A28 (-12.6991, -49.6724) -> (-11.6819, -49.5615) centre (-13.5, -37.5997) ccw
  arc A29 (-11.5682, -49.6444) -> (-11.6819, -49.5615) centre (-11.6669, -49.6604) ccw
  line L14 (-11.5682, -49.6444) -> (-11.4903, -50.1254)
  spline S14 degree 5 poles (-11.4903, -50.1254) (-11.4894, -50.131) (-11.4875, -50.1421) (-11.4842, -50.1587) (-11.479, -50.1807) (-11.4714, -50.208) (-11.463, -50.2351) (-11.4542, -50.2622) (-11.4451, -50.2891) (-11.4358, -50.3161) (-11.4263, -50.343) (-11.4165, -50.3699) (-11.4065, -50.3967) (-11.396, -50.4234) (-11.3852, -50.45) (-11.3741, -50.4766) (-11.3626, -50.503) (-11.3509, -50.5295) (-11.339, -50.5558) (-11.3269, -50.5821) (-11.3145, -50.6084) (-11.302, -50.6346) (-11.2892, -50.6608) (-11.2762, -50.6868) (-11.2629, -50.7129) (-11.2494, -50.7388) (-11.2357, -50.7648) (-11.2218, -50.7906) (-11.2078, -50.8164) (-11.1935, -50.8422) (-11.179, -50.8679) (-11.1644, -50.8935) (-11.1495, -50.9191) (-11.1345, -50.9446) (-11.1193, -50.9701) (-11.1039, -50.9955) (-11.0884, -51.0209) (-11.0726, -51.0462) (-11.0567, -51.0715) (-11.0406, -51.0967) (-11.0244, -51.1218) (-11.0079, -51.1469) (-10.9914, -51.172) (-10.9746, -51.1969) (-10.9577, -51.2219) (-10.9406, -51.2468) (-10.9234, -51.2716) (-10.906, -51.2964) (-10.8885, -51.3211) (-10.8708, -51.3457) (-10.8529, -51.3703) (-10.8349, -51.3949) (-10.8168, -51.4194) (-10.7985, -51.4438) (-10.78, -51.4682) (-10.7614, -51.4925) (-10.7427, -51.5168) (-10.7238, -51.541) (-10.7048, -51.5652) (-10.6856, -51.5893) (-10.6663, -51.6134) (-10.6468, -51.6374) (-10.6272, -51.6613) (-10.6075, -51.6852) (-10.5876, -51.709) (-10.5676, -51.7328) (-10.5475, -51.7565) (-10.5272, -51.7801) (-10.5068, -51.8037) (-10.4863, -51.8273) (-10.4656, -51.8508) (-10.4489, -51.8695) (-10.4364, -51.8835) (-10.428, -51.8929) (-10.4238, -51.8975) knots 0 0 0 0 0 0 0.01428571 0.02857143 0.04285714 0.05714286 0.07142857 0.08571429 0.1 0.11428571 0.12857143 0.14285714 0.15714286 0.17142857 0.18571429 0.2 0.21428571 0.22857143 0.24285714 0.25714286 0.27142857 0.28571429 0.3 0.31428571 0.32857143 0.34285714 0.35714286 0.37142857 0.38571429 0.4 0.41428571 0.42857143 0.44285714 0.45714286 0.47142857 0.48571429 0.5 0.51428571 0.52857143 0.54285714 0.55714286 0.57142857 0.58571429 0.6 0.61428571 0.62857143 0.64285714 0.65714286 0.67142857 0.68571429 0.7 0.71428571 0.72857143 0.74285714 0.75714286 0.77142857 0.78571429 0.8 0.81428571 0.82857143 0.84285714 0.85714286 0.87142857 0.88571429 0.9 0.91428571 0.92857143 0.94285714 0.95714286 0.97142857 0.98571429 1 1 1 1 1 1
  arc A30 (-10.4238, -51.8975) -> (-9.6419, -51.7066) centre (-13.5, -37.5997) ccw
  spline S15 degree 5 poles (-9.6419, -51.7066) (-9.6403, -51.7006) (-9.6372, -51.6884) (-9.6325, -51.6702) (-9.6264, -51.6459) (-9.6188, -51.6155) (-9.6115, -51.5852) (-9.6042, -51.5548) (-9.5971, -51.5245) (-9.5902, -51.4941) (-9.5834, -51.4638) (-9.5767, -51.4335) (-9.5702, -51.4032) (-9.5639, -51.373) (-9.5576, -51.3427) (-9.5516, -51.3125) (-9.5457, -51.2822) (-9.5399, -51.252) (-9.5343, -51.2218) (-9.5289, -51.1916) (-9.5236, -51.1615) (-9.5185, -51.1313) (-9.5135, -51.1012) (-9.5086, -51.0711) (-9.504, -51.041) (-9.4995, -51.011) (-9.4951, -50.9809) (-9.491, -50.9509) (-9.4869, -50.9209) (-9.4831, -50.8909) (-9.4794, -50.861) (-9.4759, -50.8311) (-9.4725, -50.8012) (-9.4694, -50.7713) (-9.4663, -50.7415) (-9.4635, -50.7117) (-9.4609, -50.6819) (-9.4584, -50.6521) (-9.4561, -50.6224) (-9.4539, -50.5927) (-9.452, -50.5631) (-9.4502, -50.5334) (-9.4487, -50.5039) (-9.4473, -50.4743) (-9.4461, -50.4448) (-9.4451, -50.4153) (-9.4443, -50.3859) (-9.4437, -50.3565) (-9.4433, -50.3272) (-9.4431, -50.2979) (-9.4431, -50.2686) (-9.4433, -50.2394) (-9.4438, -50.2102) (-9.4445, -50.1811) (-9.4454, -50.1521) (-9.4465, -50.1231) (-9.4479, -50.0942) (-9.4495, -50.0653) (-9.4512, -50.0364) (-9.4533, -50.0076) (-9.4556, -49.9789) (-9.4583, -49.9503) (-9.4613, -49.9218) (-9.4648, -49.8934) (-9.4685, -49.8651) (-9.4725, -49.8368) (-9.4766, -49.8086) (-9.481, -49.7804) (-9.4856, -49.7524) (-9.4907, -49.7245) (-9.4965, -49.6968) (-9.502, -49.6748) (-9.5067, -49.6585) (-9.5101, -49.6478) (-9.5119, -49.6424) knots -1 -1 -1 -1 -1 -1 -0.98571429 -0.97142857 -0.95714286 -0.94285714 -0.92857143 -0.91428571 -0.9 -0.88571429 -0.87142857 -0.85714286 -0.84285714 -0.82857143 -0.81428571 -0.8 -0.78571429 -0.77142857 -0.75714286 -0.74285714 -0.72857143 -0.71428571 -0.7 -0.68571429 -0.67142857 -0.65714286 -0.64285714 -0.62857143 -0.61428571 -0.6 -0.58571429 -0.57142857 -0.55714286 -0.54285714 -0.52857143 -0.51428571 -0.5 -0.48571429 -0.47142857 -0.45714286 -0.44285714 -0.42857143 -0.41428571 -0.4 -0.38571429 -0.37142857 -0.35714286 -0.34285714 -0.32857143 -0.31428571 -0.3 -0.28571429 -0.27142857 -0.25714286 -0.24285714 -0.22857143 -0.21428571 -0.2 -0.18571429 -0.17142857 -0.15714286 -0.14285714 -0.12857143 -0.11428571 -0.1 -0.08571429 -0.07142857 -0.05714286 -0.04285714 -0.02857143 -0.01428571 0 0 0 0 0 0
  line L15 (-9.5119, -49.6424) -> (-9.6645, -49.1797)
  arc A31 (-9.6017, -49.0537) -> (-9.6645, -49.1797) centre (-9.5695, -49.1484) ccw
  arc A32 (-9.6017, -49.0537) -> (-8.6479, -48.6834) centre (-13.5, -37.5997) ccw
  arc A33 (-8.5166, -48.734) -> (-8.6479, -48.6834) centre (-8.6078, -48.775) ccw
  line L16 (-8.5166, -48.734) -> (-8.3169, -49.1784)
  spline S16 degree 5 poles (-8.3169, -49.1784) (-8.3146, -49.1836) (-8.3099, -49.1939) (-8.3024, -49.2091) (-8.2916, -49.229) (-8.2773, -49.2534) (-8.2622, -49.2774) (-8.2466, -49.3012) (-8.2308, -49.3249) (-8.2149, -49.3485) (-8.1987, -49.3721) (-8.1824, -49.3955) (-8.1657, -49.4188) (-8.1487, -49.4419) (-8.1314, -49.4648) (-8.1138, -49.4876) (-8.0958, -49.5102) (-8.0777, -49.5327) (-8.0593, -49.555) (-8.0408, -49.5773) (-8.0221, -49.5995) (-8.0032, -49.6216) (-7.9841, -49.6435) (-7.9647, -49.6653) (-7.9452, -49.687) (-7.9255, -49.7086) (-7.9055, -49.7301) (-7.8854, -49.7515) (-7.8651, -49.7728) (-7.8447, -49.794) (-7.8241, -49.815) (-7.8033, -49.836) (-7.7823, -49.8569) (-7.7612, -49.8777) (-7.7399, -49.8983) (-7.7185, -49.9189) (-7.6969, -49.9394) (-7.6751, -49.9598) (-7.6532, -49.98) (-7.6311, -50.0002) (-7.6089, -50.0203) (-7.5866, -50.0403) (-7.5641, -50.0602) (-7.5414, -50.08) (-7.5186, -50.0997) (-7.4957, -50.1193) (-7.4726, -50.1388) (-7.4494, -50.1583) (-7.4261, -50.1776) (-7.4026, -50.1968) (-7.379, -50.216) (-7.3553, -50.2351) (-7.3314, -50.254) (-7.3074, -50.2729) (-7.2833, -50.2917) (-7.259, -50.3104) (-7.2346, -50.329) (-7.2101, -50.3475) (-7.1855, -50.3659) (-7.1607, -50.3842) (-7.1358, -50.4024) (-7.1108, -50.4206) (-7.0857, -50.4386) (-7.0605, -50.4566) (-7.0351, -50.4745) (-7.0096, -50.4922) (-6.9841, -50.5099) (-6.9583, -50.5275) (-6.9325, -50.5451) (-6.9066, -50.5625) (-6.8805, -50.5798) (-6.8596, -50.5936) (-6.8439, -50.6039) (-6.8334, -50.6108) (-6.8281, -50.6142) knots 0 0 0 0 0 0 0.01428571 0.02857143 0.04285714 0.05714286 0.07142857 0.08571429 0.1 0.11428571 0.12857143 0.14285714 0.15714286 0.17142857 0.18571429 0.2 0.21428571 0.22857143 0.24285714 0.25714286 0.27142857 0.28571429 0.3 0.31428571 0.32857143 0.34285714 0.35714286 0.37142857 0.38571429 0.4 0.41428571 0.42857143 0.44285714 0.45714286 0.47142857 0.48571429 0.5 0.51428571 0.52857143 0.54285714 0.55714286 0.57142857 0.58571429 0.6 0.61428571 0.62857143 0.64285714 0.65714286 0.67142857 0.68571429 0.7 0.71428571 0.72857143 0.74285714 0.75714286 0.77142857 0.78571429 0.8 0.81428571 0.82857143 0.84285714 0.85714286 0.87142857 0.88571429 0.9 0.91428571 0.92857143 0.94285714 0.95714286 0.97142857 0.98571429 1 1 1 1 1 1
  arc A34 (-6.8281, -50.6142) -> (-6.1222, -50.2274) centre (-13.5, -37.5997) ccw
  spline S17 degree 5 poles (-6.1222, -50.2274) (-6.1223, -50.2211) (-6.1224, -50.2086) (-6.1226, -50.1898) (-6.1229, -50.1647) (-6.1235, -50.1334) (-6.1243, -50.1022) (-6.1251, -50.071) (-6.1261, -50.0399) (-6.1273, -50.0088) (-6.1285, -49.9777) (-6.1299, -49.9467) (-6.1315, -49.9158) (-6.1332, -49.8849) (-6.135, -49.8541) (-6.137, -49.8233) (-6.1391, -49.7926) (-6.1414, -49.7619) (-6.1438, -49.7313) (-6.1463, -49.7007) (-6.149, -49.6702) (-6.1519, -49.6398) (-6.1549, -49.6094) (-6.158, -49.579) (-6.1613, -49.5488) (-6.1647, -49.5186) (-6.1683, -49.4884) (-6.172, -49.4584) (-6.1759, -49.4283) (-6.1799, -49.3984) (-6.1841, -49.3685) (-6.1885, -49.3387) (-6.193, -49.309) (-6.1976, -49.2793) (-6.2025, -49.2497) (-6.2074, -49.2202) (-6.2126, -49.1907) (-6.2179, -49.1613) (-6.2233, -49.132) (-6.229, -49.1028) (-6.2348, -49.0736) (-6.2407, -49.0446) (-6.2469, -49.0156) (-6.2532, -48.9867) (-6.2597, -48.9579) (-6.2663, -48.9292) (-6.2732, -48.9005) (-6.2802, -48.872) (-6.2874, -48.8435) (-6.2948, -48.8152) (-6.3024, -48.7869) (-6.3101, -48.7588) (-6.3181, -48.7307) (-6.3263, -48.7028) (-6.3348, -48.675) (-6.3434, -48.6473) (-6.3522, -48.6197) (-6.3612, -48.5922) (-6.3703, -48.5648) (-6.3798, -48.5375) (-6.3894, -48.5104) (-6.3994, -48.4834) (-6.4098, -48.4567) (-6.4204, -48.4301) (-6.4314, -48.4037) (-6.4425, -48.3774) (-6.4538, -48.3513) (-6.4653, -48.3252) (-6.477, -48.2993) (-6.4892, -48.2736) (-6.502, -48.2484) (-6.513, -48.2286) (-6.5218, -48.2141) (-6.5278, -48.2046) (-6.5309, -48.1999) knots -1 -1 -1 -1 -1 -1 -0.98571429 -0.97142857 -0.95714286 -0.94285714 -0.92857143 -0.91428571 -0.9 -0.88571429 -0.87142857 -0.85714286 -0.84285714 -0.82857143 -0.81428571 -0.8 -0.78571429 -0.77142857 -0.75714286 -0.74285714 -0.72857143 -0.71428571 -0.7 -0.68571429 -0.67142857 -0.65714286 -0.64285714 -0.62857143 -0.61428571 -0.6 -0.58571429 -0.57142857 -0.55714286 -0.54285714 -0.52857143 -0.51428571 -0.5 -0.48571429 -0.47142857 -0.45714286 -0.44285714 -0.42857143 -0.41428571 -0.4 -0.38571429 -0.37142857 -0.35714286 -0.34285714 -0.32857143 -0.31428571 -0.3 -0.28571429 -0.27142857 -0.25714286 -0.24285714 -0.22857143 -0.21428571 -0.2 -0.18571429 -0.17142857 -0.15714286 -0.14285714 -0.12857143 -0.11428571 -0.1 -0.08571429 -0.07142857 -0.05714286 -0.04285714 -0.02857143 -0.01428571 0 0 0 0 0 0
  line L17 (-6.5309, -48.1999) -> (-6.798, -47.7924)
  arc A35 (-6.77, -47.6545) -> (-6.798, -47.7924) centre (-6.7144, -47.7376) ccw
  arc A36 (-6.77, -47.6545) -> (-5.9446, -47.0499) centre (-13.5, -37.5997) ccw
  arc A37 (-5.8046, -47.0648) -> (-5.9446, -47.0499) centre (-5.8821, -47.128) ccw
  line L18 (-5.8046, -47.0648) -> (-5.4968, -47.4424)
  spline S18 degree 5 poles (-5.4968, -47.4424) (-5.4932, -47.4468) (-5.4859, -47.4555) (-5.4747, -47.4682) (-5.4592, -47.4847) (-5.439, -47.5045) (-5.4182, -47.5238) (-5.3971, -47.5428) (-5.3757, -47.5616) (-5.3541, -47.5803) (-5.3325, -47.5989) (-5.3106, -47.6173) (-5.2885, -47.6354) (-5.2661, -47.6534) (-5.2434, -47.671) (-5.2205, -47.6884) (-5.1973, -47.7056) (-5.174, -47.7227) (-5.1505, -47.7395) (-5.1268, -47.7562) (-5.103, -47.7728) (-5.079, -47.7892) (-5.0548, -47.8055) (-5.0305, -47.8216) (-5.006, -47.8375) (-4.9814, -47.8532) (-4.9566, -47.8688) (-4.9316, -47.8843) (-4.9065, -47.8996) (-4.8813, -47.9148) (-4.8559, -47.9298) (-4.8304, -47.9447) (-4.8048, -47.9594) (-4.779, -47.974) (-4.7531, -47.9885) (-4.727, -48.0028) (-4.7009, -48.017) (-4.6746, -48.031) (-4.6482, -48.0449) (-4.6216, -48.0587) (-4.595, -48.0724) (-4.5682, -48.0859) (-4.5413, -48.0993) (-4.5143, -48.1126) (-4.4872, -48.1257) (-4.46, -48.1387) (-4.4327, -48.1516) (-4.4052, -48.1644) (-4.3777, -48.177) (-4.35, -48.1895) (-4.3222, -48.2019) (-4.2944, -48.2141) (-4.2664, -48.2263) (-4.2383, -48.2383) (-4.2102, -48.2502) (-4.1819, -48.262) (-4.1535, -48.2736) (-4.1251, -48.2851) (-4.0965, -48.2966) (-4.0679, -48.3079) (-4.0391, -48.319) (-4.0103, -48.3301) (-3.9813, -48.341) (-3.9523, -48.3518) (-3.9232, -48.3625) (-3.894, -48.3731) (-3.8647, -48.3836) (-3.8353, -48.3939) (-3.8058, -48.4042) (-3.7763, -48.4143) (-3.7466, -48.4243) (-3.7228, -48.4322) (-3.7049, -48.4381) (-3.693, -48.442) (-3.687, -48.4439) knots 0 0 0 0 0 0 0.01428571 0.02857143 0.04285714 0.05714286 0.07142857 0.08571429 0.1 0.11428571 0.12857143 0.14285714 0.15714286 0.17142857 0.18571429 0.2 0.21428571 0.22857143 0.24285714 0.25714286 0.27142857 0.28571429 0.3 0.31428571 0.32857143 0.34285714 0.35714286 0.37142857 0.38571429 0.4 0.41428571 0.42857143 0.44285714 0.45714286 0.47142857 0.48571429 0.5 0.51428571 0.52857143 0.54285714 0.55714286 0.57142857 0.58571429 0.6 0.61428571 0.62857143 0.64285714 0.65714286 0.67142857 0.68571429 0.7 0.71428571 0.72857143 0.74285714 0.75714286 0.77142857 0.78571429 0.8 0.81428571 0.82857143 0.84285714 0.85714286 0.87142857 0.88571429 0.9 0.91428571 0.92857143 0.94285714 0.95714286 0.97142857 0.98571429 1 1 1 1 1 1
  arc A38 (-3.687, -48.4439) -> (-3.1053, -47.8876) centre (-13.5, -37.5997) ccw